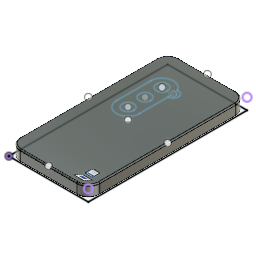
PIP-PRoS (Autodesk Fusion 360 archive; units mm, degrees)
design "Celular"
Autodesk Fusion 360 part; units mm, degrees
sketch "Esboço1" plane through (0, 0, 0) normal (0, 0, 1) x (1, 0, 0)
  line L0 (0, 0) -> (70, 0)
  line L1 (70, 0) -> (70, 140)
  line L2 (70, 140) -> (0, 140)
  line L3 (0, 140) -> (0, 0)
  circle A0 centre (15, 120) radius 5
  circle A1 centre (15, 105) radius 5
  circle A2 centre (15, 90) radius 5
  line L4 (5, 120) -> (5, 90)
  arc A3 (5, 90) -> (25, 90) centre (15, 90) ccw
  circle A4 centre (25, 120) radius 2.5
  arc A5 (25, 115.5) -> (23.9875, 124.3846) centre (25, 120) ccw
  line L5 (25, 120) -> (25, 117.5)
  line L6 (25, 115.5) -> (25, 90)
  arc A6 (25, 120) -> (24.6875, 122.4804) centre (15, 120) ccw
  arc A7 (23.9875, 124.3846) -> (5, 120) centre (15, 120) ccw
  dimension "d1" = 70
  dimension "d2" = 140
  dimension "d3" = 10
  dimension "d4" = 10
  dimension "d5" = 10
  dimension "d8" = 5
  constraint horizontal L0
  constraint vertical L1
  constraint horizontal L2
  constraint vertical L3
  constraint coincident L0.start L3.end
  constraint tangent A3 L5
  constraint parallel L3 L5
  constraint tangent L4 A3
  constraint parallel L4 L5
  constraint concentric A0 A6
  constraint concentric A2 A3
  constraint coincident A4.centre L5
  constraint coincident A4.centre A5.centre
  constraint concentric A4 A5
  constraint coincident A5.end A6
  constraint coincident A5.start L5
  constraint coincident A4 L5.end
  constraint collinear L5 L6
  constraint coincident A4 A6.end
  constraint concentric A6 A7
  measures "d1" distance of L0.start L0.end
  measures "d2" distance of L0.start L2.end
  measures "d3" diameter of A0
  measures "d4" diameter of A1
  measures "d5" diameter of A2
  measures "d8" diameter of A4
extrude "Extrusão1" add sketch "Esboço1" along normal blind 10 contours L0 L1 L2 L3 | A0 | A1 | A2 | L4 A3 A5 L6 A7 | A4 L5 A6 | A4 L5 A6
extrude "Extrusão2" add sketch "Esboço1" against normal blind 2 contours L4 A3 A5 L6 A7
fillet "Arredondamento1" radius 1 4 edges at (70, 70, 10) (35, 0, 10) (0, 70, 10) (35, 140, 10)
fillet "Arredondamento2" radius 1 4 edges at (70, 70, 0) (35, 0, 0) (0, 70, 0) (35, 140, 0)
fillet "Arredondamento3" radius 10 12 edges at (69.7071, 0.2929, 0.2929) (70, 0, 5) (69.7071, 0.2929, 9.7071) (69.7071, 139.7071, 0.2929) (70, 140, 5) (69.7071, 139.7071, 9.7071) (0.2929, 139.7071, 0.2929) (0, 140, 5) (0.2929, 139.7071, 9.7071) (0.2929, 0.2929, 0.2929) (0, 0, 5) (0.2929, 0.2929, 9.7071)
sketch "Esboço2" plane through (0, 0, 10) normal (0, 0, 1) x (-1, 0, 0)
  arc A0 (-1, -10) -> (-10, -1) centre (-10, -10) ccw
  line L0 (-10, -1) -> (-60, -1)
  arc A1 (-60, -1) -> (-69, -10) centre (-60, -10) ccw
  line L1 (-69, -10) -> (-69, -130)
  arc A2 (-69, -130) -> (-60, -139) centre (-60, -130) ccw
  line L2 (-60, -139) -> (-10, -139)
  arc A3 (-10, -139) -> (-1, -130) centre (-10, -130) ccw
  line L3 (-1, -130) -> (-1, -10)
sketch "Esboço3" plane through (0, 0, 10) normal (0, 0, 1) x (-1, 0, 0)
  point P0 (0, -70)
  point P1 (-70, -70)
  point P2 (-35, -140)
  point P3 (-35, 0)
  point P4 (-70, -140)
  point P5 (-70, 0)
  point P6 (-35, -70)
  dimension "d20" = 35
  dimension "d21" = 35
  measures "d20" distance of P2 P4
  measures "d21" distance of P3 P5
